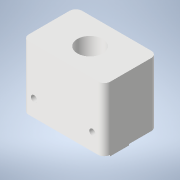
# Autodesk Inventor part: Soporte placa 2.0
Saved by Autodesk Inventor 2020.3 (Build 243373000, 373)
## iProperties
Created: 2020-05-18
Part Number: Soporte placa 2.0
Material: Genérico
Document SubType Name: Modeling
Designer: javic
Density: 1 g/cm^3
Appearance: Valor por defecto
Mass: 1.00664 g
Surface Area: 7.35186 cm^2
Volume: 1.00664 cm^3
Author: javic
Autodesk Inventor part; units mm, degrees
ref_plane "YZ Plane" through (0, 0, 0) normal (1, 0, 0) x (0, 1, 0)
ref_plane "XZ Plane" through (0, 0, 0) normal (0, 1, 0) x (-1, 0, 0)
ref_plane "XY Plane" through (0, 0, 0) normal (0, 0, 1) x (1, 0, 0)
sketch "Boceto1" plane through (0, 0, 0) normal (0, 1, 0) x (-1, 0, 0)
  line L0 (0, 0) -> (0, -8.5)
  line L1 (0, -8.5) -> (13, -8.5)
  line L2 (13, -8.5) -> (13, 0)
  line L3 (13, 0) -> (0, 0)
  circle A0 centre (6.5, -4.25) radius 0.9
  dimension "d0" = 8.5
  dimension "d1" = 13
  dimension "d2" = 1.8
  dimension "d13" = 4.25
  constraints: 8 end point, 3 perpendicular, 1 centre point, 1 vertical
  measures "d0" distance of L0.start L0.end
  measures "d1" distance of L0.end L1.end
  measures "d2" diameter of A0
  measures "d13" distance from line of L3 A0.centre
extrude "Extrusión1" add sketch "Boceto1" along normal blind 10.06
sketch "Boceto2" plane through (0, 10.06, 0) normal (0, 1, 0) x (1, 0, 0)
  circle A0 centre (-6.5, 4.25) radius 0.9 projected
  point P0 (0, 0)
  constraints: 3 coincident
hole "Agujero1" at (-6.5, 10.06, -4.25) direction (0, -1, 0) diameter 4 depth 7.06
fillet "Empalme1" radius 1 4 edges at (0, 5.03, 0) (0, 5.03, -8.5) (-13, 5.03, 0) (-13, 5.03, -8.5)
sketch "Boceto3" plane through (0, 0, 0) normal (0, -1, 0) x (1, 0, 0)
  line L0 (-1.8, -5.75) -> (-3.8, -5.75)
  line L1 (-3.8, -5.75) -> (-3.8, -2.75)
  line L2 (-3.8, -2.75) -> (-1.8, -2.75)
  line L3 (-1.8, -2.75) -> (-1.8, -5.75)
  line L4 (0, -1) -> (0, -7.5) projected
  line L5 (-1, -8.5) -> (-12, -8.5) projected
  line L6 (-9.2, -5.75) -> (-11.2, -5.75)
  line L7 (-11.2, -5.75) -> (-11.2, -2.75)
  line L8 (-11.2, -2.75) -> (-9.2, -2.75)
  line L9 (-9.2, -2.75) -> (-9.2, -5.75)
  line L10 (-12, 0) -> (-1, 0) projected
  line L11 (-13, -7.5) -> (-13, -1) projected
  point P0 (0, 0)
  dimension "d14" = 2
  dimension "d15" = 3
  dimension "d16" = 1.8
  dimension "d17" = 2.75
  dimension "d18" = 2
  dimension "d19" = 3
  dimension "d20" = 2.75
  dimension "d21" = 1.8
  constraints: 16 end point, 4 parallel, 2 horizontal, 2 perpendicular
  measures "d14" distance of L1.end L2.end
  measures "d15" distance of L0.end L1.end
  measures "d16" distance between parallel lines of L4 L3
  measures "d17" distance between parallel lines of L5 L0
  measures "d18" distance of L7.end L8.end
  measures "d19" distance of L6.end L7.end
  measures "d20" distance between parallel lines of L10 L8
  measures "d21" distance between parallel lines of L11 L7
extrude "Extrusión2" add sketch "Boceto3" along normal blind 2
sketch "Boceto4" plane through (-12, 0, 0) normal (0, 0, 1) x (1, 0, 0)
  circle A0 centre (1.25, 4) radius 0.5
  circle A1 centre (9.75, 4) radius 0.5
  line L0 (-1, 10.06) -> (-1, 0) projected
  line L1 (12, 0) -> (12, 10.06) projected
  line L2 (0, 0) -> (11, 0) projected
  dimension "d24" = 1
  dimension "d25" = 1
  dimension "d26" = 2.25
  dimension "d27" = 2.25
  dimension "d28" = 4
  dimension "d29" = 4
  constraints: 2 centre point
  measures "d24" diameter of A0
  measures "d25" diameter of A1
  measures "d26" distance from line of L0 A0.centre
  measures "d27" distance from line of L1 A1.centre
  measures "d28" distance from line of L2 A0.centre
  measures "d29" distance from line of L2 A1.centre
hole "Agujero2" at (-10.75, 4, 0) at (-2.25, 4, 0) direction (0, 0, -1) diameter 1 end through all
